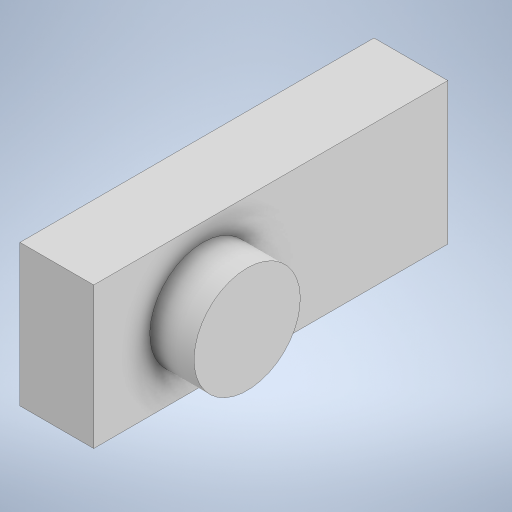
# Autodesk Inventor part: Cámara
Saved by Autodesk Inventor 2024.1 (Build 281209000, 209)
## iProperties
Created: 2023-08-13
Part Number: Cámara
Material: Genérico
Document SubType Name: Modeling
Designer: Det-Pc
Density: 1 g/cm^3
Appearance: Valor por defecto
Author: Det-Pc
Autodesk Inventor part; units mm, degrees
ref_plane "YZ Plane" through (0, 0, 0) normal (1, 0, 0) x (0, 1, 0)
ref_plane "XZ Plane" through (0, 0, 0) normal (0, 1, 0) x (-1, 0, 0)
ref_plane "XY Plane" through (0, 0, 0) normal (0, 0, 1) x (1, 0, 0)
sketch "Boceto1" plane through (0, 0, 0) normal (1, 0, 0) x (0, 1, 0)
  line L0 (12, 30) -> (-12, 30)
  line L1 (-12, 30) -> (-12, -30)
  line L2 (-12, -30) -> (12, -30)
  line L3 (12, -30) -> (12, 30)
  circle A0 centre (0, 11.5) radius 9
  point P0 (0, 0)
  point P1 (12, 0)
  point P2 (0, -30)
  dimension "d0" = 60
  dimension "d1" = 24
  dimension "d2" = 18
  dimension "d3" = 18.5
  constraints: 8 end point, 2 midpoint, 2 parallel, 2 vertical alignment, 1 centre point, 1 horizontal, 1 horizontal alignment, 1 perpendicular
  measures "d0" distance of L2.end L0.start
  measures "d1" distance of L1.end L2.end
  measures "d2" diameter of A0
  measures "d3" distance from line of L0 A0.centre
extrude "Extrusión1" add sketch "Boceto1" along normal blind 20 contours A0
extrude "Extrusión2" add sketch "Boceto1" along normal blind 12.5
